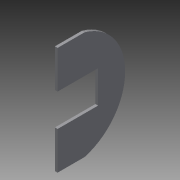
# Autodesk Inventor part: beam
Saved by Autodesk Inventor 2015 (Build 190159000, 159)
## iProperties
Created: 2014-08-30
Part Number: beam
Material: Generic
Document SubType Name: Modeling
Designer: shohei
Density: 1 g/cm^3
Appearance: Default
Author: shohei
Autodesk Inventor part; units mm, degrees
ref_plane "YZ Plane" through (0, 0, 0) normal (1, 0, 0) x (0, 1, 0)
ref_plane "XZ Plane" through (0, 0, 0) normal (0, 1, 0) x (-1, 0, 0)
ref_plane "XY Plane" through (0, 0, 0) normal (0, 0, 1) x (1, 0, 0)
sketch "Sketch1" plane through (0, 0, 0) normal (1, 0, 0) x (0, 1, 0)
  line L0 (48.3789, 0) -> (148.3789, 0)
  line L1 (248.3789, -333.1357) -> (248.3789, -336.1798)
  line L2 (148.3789, -400) -> (48.3789, -400)
  line L3 (48.3789, -400) -> (48.3789, 0)
  line L4 (198.3789, -260) -> (48.3789, -260)
  line L5 (48.3789, -260) -> (48.3789, -140)
  line L6 (48.3789, -140) -> (198.3789, -140)
  line L7 (198.3789, -140) -> (198.3789, -260)
  line L8 (-98.7773, -200) -> (409.3156, -200)
  arc A0 (298.3789, -200) -> (148.3789, 0) centre (92.075, -198.478) ccw
  arc A1 (148.3789, -400) -> (298.3789, -200) centre (92.075, -201.522) ccw
  point P0 (248.3789, -63.8202)
  point P1 (248.3789, -200)
  dimension "d11" = 120
  dimension "d12" = 150
  dimension "d13" = 50
  dimension "d14" = 140
  dimension "d18" = 200
  dimension "d19" = 200
  dimension "d20" = 50
  dimension "d21" = 100
  dimension "d23" = 400
  constraints: 18 end point, 7 point on circle, 3 horizontal, 3 parallel, 2 centre point, 2 perpendicular, 2 symmetric about line, 1 coincident, 1 point on line, 1 other
  measures "d11" distance of L4.end L5.end
  measures "d12" distance of L5.end L6.end
  measures "d13" distance between parallel lines of L1 L7
  measures "d14" distance between parallel lines of L0 L6
  measures "d18" distance between parallel lines of L0 L8
  measures "d19" distance from line of point (248.379, -200) L0
  measures "d20" distance of point (248.379, -200) A0.start
  measures "d21" distance of L0.start L0.end
  measures "d23" distance of L0.start point (48.379, -400)
extrude "Extrusion1" add sketch "Sketch1" along normal blind 10 contours L0 A0 L8 L7 L6 L3 | A1 L2 L3 L4 L7 L8
body "Solid1"
